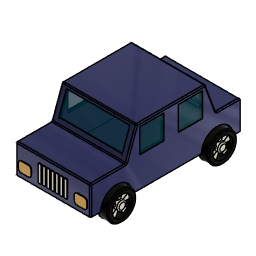
P7 (Autodesk Fusion 360 design; units mm, degrees)
Autodesk Fusion 360 part; units mm, degrees
note: some values were not read from the file. Chosen so that the rebuilt part matches the saved one: which bodies a step acts on. Set by a fixed rule: which sketch regions a step uses.
sketch "Sketch1" plane through (0, 0, 0) normal (1, 0, 0) x (0, 1, 0)
  line L0 (-140, 0) -> (120, 0)
  line L1 (120, 0) -> (120, 50)
  line L2 (120, 50) -> (78.1985, 50)
  line L3 (78.1985, 50) -> (60, 100)
  line L4 (60, 100) -> (-60, 100)
  line L5 (-60, 100) -> (-78.1985, 50)
  line L6 (-78.1985, 50) -> (-140, 50)
  line L7 (-140, 50) -> (-140, 0)
  line L8 (0, 0) -> (0, 100) construction
  dimension "d1" = 120
  dimension "d2" = 50
  dimension "d3" = 100
  dimension "d4" = 120
  dimension "d5" = 260
  dimension "d6" = 110
  dimension "d7" = 110
  constraint horizontal L0
  constraint perpendicular L1 L2
  constraint coincident L8.start origin
  constraint midpoint L4 L8.end
  constraint perpendicular L4 L8
  constraint symmetric L3 L5 L8
  constraint collinear L2 L6
  constraint vertical L7
  constraint perpendicular L6 L7
  constraint coincident L8.start L0
  measures "d1" distance of L3.end L4.end
  measures "d2" distance of L0.end L1.end
  measures "d3" distance of L0 L3.end
  measures "d4" horizontal distance of L8.start L0.end
  measures "d5" distance of L0.start L0.end
  measures "d6" angle of L5 L6
  measures "d7" angle of L2 L3
extrude "Extrude1" add sketch "Sketch1" along normal mid plane 130 makes body 1
shell "Shell1" thickness 5 removed faces 0 bodies 1
sketch "Sketch2" plane through (65, 0, 0) normal (1, 0, 0) x (0, 1, 0)
  line L0 (-140, 50) -> (-140, 0)
  line L1 (-140, 0) -> (120, 0)
  line L2 (120, 0) -> (120, 50)
  line L3 (120, 50) -> (78.1985, 50)
  line L4 (78.1985, 50) -> (60, 100)
  line L5 (60, 100) -> (-60, 100)
  line L6 (-60, 100) -> (-78.1985, 50)
  line L7 (-78.1985, 50) -> (-140, 50)
  line L8 (0, 0) -> (0, 100) construction
  line L9 (-12.5, 94) -> (-54.5, 94)
  line L10 (-54.5, 94) -> (-54.5, 52)
  line L11 (-54.5, 52) -> (-12.5, 52)
  line L12 (-12.5, 52) -> (-12.5, 94)
  line L13 (12.5, 52) -> (12.5, 94)
  line L14 (12.5, 94) -> (54.5, 94)
  line L15 (54.5, 94) -> (54.5, 52)
  line L16 (54.5, 52) -> (12.5, 52)
  dimension "d16" = 42
  dimension "d17" = 42
  dimension "d18" = 12.5
  dimension "d19" = 6
  constraint coincident L8.start origin
  constraint midpoint L5 L8.end
  constraint horizontal L9
  constraint vertical L10
  constraint horizontal L11
  constraint vertical L12
  constraint symmetric L9.start L8 L13.end
  constraint symmetric L8 L9.end L14.end
  constraint symmetric L8 L10.end L15.end
  constraint symmetric L8 L11.end L13.start
  measures "d16" distance of L9.start L9.end
  measures "d17" distance of L9.start L11.end
  measures "d18" horizontal distance of L9.start L8.end
  measures "d19" vertical distance of L5.end L9.end
extrude "Extrude2" cut sketch "Sketch2" against normal blind 130 contours L9 L10 L11 L12 | L13 L14 L15 L16 bodies 1
sketch "Sketch3" plane through (0, 0, 0) normal (0, 1, 0) x (1, 0, 0)
  line L0 (55, -95) -> (-55, -95)
  line L1 (-55, -95) -> (-55, -55)
  line L2 (-55, -55) -> (55, -55)
  line L3 (55, -55) -> (55, -95)
  line L4 (-65, -100) -> (65, -100)
  line L5 (0, 0) -> (0, -100) construction
  dimension "d24" = 5
  dimension "d25" = 40
  dimension "d26" = 110
  constraint horizontal L0
  constraint vertical L1
  constraint horizontal L2
  constraint vertical L3
  constraint coincident L5.start origin
  constraint midpoint L4 L5.end
  constraint symmetric L1 L3 L5
  measures "d24" distance of L0.end L4
  measures "d25" distance of L0.end L1.end
  measures "d26" distance of L0.start L0.end
extrude "Extrude3" cut sketch "Sketch3" along normal mid plane 150 bodies 1
sketch "Sketch4" plane through (65, 0, 0) normal (1, 0, 0) x (0, 1, 0)
  line L0 (-54.5, 94) -> (-12.5, 94)
  line L1 (-12.5, 94) -> (-12.5, 52)
  line L2 (-12.5, 52) -> (-54.5, 52)
  line L3 (-54.5, 52) -> (-54.5, 94)
  line L4 (12.5, 94) -> (54.5, 94)
  line L5 (54.5, 94) -> (54.5, 52)
  line L6 (54.5, 52) -> (12.5, 52)
  line L7 (12.5, 52) -> (12.5, 94)
  line L8 (-140, 50) -> (-140, 0)
  line L9 (-140, 0) -> (120, 0)
  line L10 (120, 0) -> (120, 50)
  line L11 (120, 50) -> (78.1985, 50)
  line L12 (78.1985, 50) -> (60, 100)
  line L13 (60, 100) -> (-60, 100)
  line L14 (-60, 100) -> (-78.1985, 50)
  line L15 (-78.1985, 50) -> (-140, 50)
  line L16 (-54.5, 94) -> (-12.5, 94)
  line L17 (-12.5, 94) -> (-12.5, 52)
  line L18 (-12.5, 52) -> (-54.5, 52)
  line L19 (-54.5, 52) -> (-54.5, 94)
  line L20 (12.5, 94) -> (54.5, 94)
  line L21 (54.5, 94) -> (54.5, 52)
  line L22 (54.5, 52) -> (12.5, 52)
  line L23 (12.5, 52) -> (12.5, 94)
  constraint horizontal L16
  constraint vertical L17
  constraint horizontal L18
  constraint vertical L19
  constraint coincident L1.end L2.start
  constraint coincident L0.start L3.end
  constraint horizontal L20
  constraint vertical L21
  constraint horizontal L22
  constraint vertical L23
  constraint coincident L5.end L6.start
  constraint coincident L4.start L7.end
extrude "Extrude4" add sketch "Sketch4" against normal blind 2 separate body contours L0 L1 L2 L3 L16 L17 L18 L19 | L4 L5 L6 L7 L20 L21 L22 L23 makes body 2 at (65, -40.5, 80) makes body 3 at (65, 40.5, 66)
mirror "Mirror1" about plane through (0, 0, 0) normal (1, 0, 0) of bodies 2 3 makes body 4 at (-65, -40.5, 80) makes body 5 at (-65, 40.5, 66)
sketch "Sketch5" plane through (0, -85.1207, 30.9814) normal (0, -0.939693, 0.34202) x (1, 0, 0)
  line L0 (55, 29.591) -> (-55, 29.591)
  line L1 (-55, 29.591) -> (-55, 68.1272)
  line L2 (-55, 68.1272) -> (55, 68.1272)
  line L3 (55, 68.1272) -> (55, 29.591)
  line L4 (-65, 20.2392) -> (65, 20.2392)
  line L5 (65, 20.2392) -> (65, 73.4481)
  line L6 (65, 73.4481) -> (-65, 73.4481)
  line L7 (-65, 73.4481) -> (-65, 20.2392)
  line L8 (-55, 29.591) -> (55, 29.591)
  line L9 (55, 29.591) -> (55, 68.1272)
  line L10 (55, 68.1272) -> (-55, 68.1272)
  line L11 (-55, 68.1272) -> (-55, 29.591)
  constraint horizontal L8
  constraint vertical L9
  constraint horizontal L10
  constraint vertical L11
  constraint coincident L2.end L3.start
  constraint coincident L0.end L1.start
extrude "Extrude5" add sketch "Sketch5" against normal blind 2 separate body contours L0 L1 L2 L3 L8 L9 L10 L11 makes body 6
mirror "Mirror2" about plane through (0, 0, 0) normal (0, 1, 0) of bodies 6 makes body 7
sketch "Sketch6" plane through (0, -140, 0) normal (0, -1, 0) x (1, 0, 0)
  line L0 (-65, 0) -> (65, 0)
  line L1 (65, 0) -> (65, 50)
  line L2 (65, 50) -> (-65, 50)
  line L3 (-65, 50) -> (-65, 0)
  line L4 (0, 0) -> (0, 50) construction
  line L5 (-54.5, 26) -> (-42.5, 26)
  line L6 (-37.5, 21) -> (-37.5, 13)
  line L7 (-42.5, 8) -> (-54.5, 8)
  line L8 (-59.5, 13) -> (-59.5, 21)
  arc A0 (-54.5, 26) -> (-59.5, 21) centre (-54.5, 21) ccw
  arc A1 (-37.5, 21) -> (-42.5, 26) centre (-42.5, 21) ccw
  arc A2 (-59.5, 13) -> (-54.5, 8) centre (-54.5, 13) ccw
  arc A3 (-42.5, 8) -> (-37.5, 13) centre (-42.5, 13) ccw
  arc A4 (42.5, 26) -> (37.5, 21) centre (42.5, 21) ccw
  line L9 (54.5, 26) -> (42.5, 26)
  arc A5 (59.5, 21) -> (54.5, 26) centre (54.5, 21) ccw
  line L10 (59.5, 13) -> (59.5, 21)
  arc A6 (54.5, 8) -> (59.5, 13) centre (54.5, 13) ccw
  line L11 (42.5, 8) -> (54.5, 8)
  arc A7 (37.5, 13) -> (42.5, 8) centre (42.5, 13) ccw
  line L12 (37.5, 21) -> (37.5, 13)
  dimension "d37" = 5
  dimension "d38" = 5
  dimension "d39" = 5
  dimension "d40" = 5
  dimension "d41" = 18
  dimension "d42" = 22
  dimension "d43" = 8
  dimension "d44" = 37.5
  constraint coincident L4.start origin
  constraint midpoint L2 L4.end
  constraint horizontal L5
  constraint vertical L6
  constraint horizontal L7
  constraint vertical L8
  constraint tangent L8 A0
  constraint tangent L5 A0
  constraint tangent L5 A1
  constraint tangent L6 A1
  constraint tangent L8 A2
  constraint tangent L7 A2
  constraint tangent L7 A3
  constraint tangent L6 A3
  constraint symmetric L4 L8.end A5.start
  constraint symmetric L4 L5.start L9.start
  constraint symmetric L4 A0 A5
  constraint symmetric L4 L5.end A4.start
  constraint symmetric L4 L6.start A4.end
  constraint symmetric L4 A1 A4
  constraint symmetric L4 L8.start L10.start
  constraint symmetric L4 L7.end A6.start
  constraint symmetric L4 A2 A6
  constraint symmetric L4 L7.start L11.start
  constraint symmetric L4 L6.end A7.start
  constraint symmetric L4 A3 A7
  measures "d37" radius of A0
  measures "d38" radius of A1
  measures "d39" radius of A2
  measures "d40" radius of A3
  measures "d41" distance of L5 L7
  measures "d42" distance of L6 L8
  measures "d43" distance of L0 L7
  measures "d44" distance of L4 L6
extrude "Extrude6" add sketch "Sketch6" along normal blind 1 contours L5 L6 L7 L8 A0 A1 A2 A3 | A4 L9 A5 L10 A6 L11 A7 L12 bodies 1
sketch "Sketch7" plane through (0, 120, 0) normal (0, 1, 0) x (-1, 0, 0)
  line L0 (65, 50) -> (-65, 50)
  line L1 (-65, 50) -> (-65, 0)
  line L2 (-65, 0) -> (65, 0)
  line L3 (65, 0) -> (65, 50)
  line L4 (-54.5, 26) -> (-42.5, 26)
  line L5 (-37.5, 21) -> (-37.5, 13)
  line L6 (-42.5, 8) -> (-54.5, 8)
  line L7 (-59.5, 13) -> (-59.5, 21)
  arc A0 (-54.5, 26) -> (-59.5, 21) centre (-54.5, 21) ccw
  arc A1 (-59.5, 13) -> (-54.5, 8) centre (-54.5, 13) ccw
  arc A2 (-42.5, 8) -> (-37.5, 13) centre (-42.5, 13) ccw
  arc A3 (-37.5, 21) -> (-42.5, 26) centre (-42.5, 21) ccw
  line L8 (0, 0) -> (0, 50) construction
  arc A4 (42.5, 26) -> (37.5, 21) centre (42.5, 21) ccw
  line L9 (54.5, 26) -> (42.5, 26)
  arc A5 (59.5, 21) -> (54.5, 26) centre (54.5, 21) ccw
  line L10 (59.5, 13) -> (59.5, 21)
  arc A6 (54.5, 8) -> (59.5, 13) centre (54.5, 13) ccw
  line L11 (42.5, 8) -> (54.5, 8)
  arc A7 (37.5, 13) -> (42.5, 8) centre (42.5, 13) ccw
  line L12 (37.5, 21) -> (37.5, 13)
  dimension "d47" = 5
  dimension "d48" = 22
  dimension "d49" = 37.5
  dimension "d50" = 18
  dimension "d51" = 8
  constraint horizontal L4
  constraint vertical L5
  constraint horizontal L6
  constraint vertical L7
  constraint tangent L4 A0
  constraint tangent L7 A0
  constraint tangent L6 A1
  constraint tangent L7 A1
  constraint equal A0 A1
  constraint tangent L6 A2
  constraint tangent L5 A2
  constraint equal A0 A2
  constraint tangent L4 A3
  constraint tangent L5 A3
  constraint equal A0 A3
  constraint coincident L8.start origin
  constraint midpoint L0 L8.end
  constraint symmetric L4.start L8 L9.start
  constraint symmetric L7.end L8 A5.start
  constraint symmetric A0 L8 A5
  constraint symmetric L6.end L8 A6.start
  constraint symmetric L7.start L8 L10.start
  constraint symmetric A1 L8 A6
  constraint symmetric L6.start L8 L11.start
  constraint symmetric L5.end L8 A7.start
  constraint symmetric A2 L8 A7
  constraint symmetric L4.end L8 A4.start
  constraint symmetric L5.start L8 A4.end
  constraint symmetric A3 L8 A4
  measures "d47" radius of A0
  measures "d48" distance of L5 L7
  measures "d49" distance of L5 L8
  measures "d50" distance of L4 L6
  measures "d51" distance of L2 L6
extrude "Extrude7" add sketch "Sketch7" along normal blind 1 contours L4 L5 L6 L7 A0 A1 A2 A3 | A4 L9 A5 L10 A6 L11 A7 L12 bodies 1
sketch "Sketch8" plane through (0, -140, 0) normal (0, -1, 0) x (1, 0, 0)
  arc A0 (42.5, 26) -> (37.5, 21) centre (42.5, 21) ccw
  line L0 (42.5, 26) -> (54.5, 26)
  arc A1 (59.5, 21) -> (54.5, 26) centre (54.5, 21) ccw
  line L1 (59.5, 21) -> (59.5, 13)
  arc A2 (54.5, 8) -> (59.5, 13) centre (54.5, 13) ccw
  line L2 (54.5, 8) -> (42.5, 8)
  arc A3 (37.5, 13) -> (42.5, 8) centre (42.5, 13) ccw
  line L3 (37.5, 13) -> (37.5, 21)
  line L4 (-59.5, 13) -> (-59.5, 21)
  arc A4 (-54.5, 26) -> (-59.5, 21) centre (-54.5, 21) ccw
  line L5 (-54.5, 26) -> (-42.5, 26)
  arc A5 (-37.5, 21) -> (-42.5, 26) centre (-42.5, 21) ccw
  line L6 (-37.5, 21) -> (-37.5, 13)
  arc A6 (-42.5, 8) -> (-37.5, 13) centre (-42.5, 13) ccw
  line L7 (-42.5, 8) -> (-54.5, 8)
  arc A7 (-59.5, 13) -> (-54.5, 8) centre (-54.5, 13) ccw
  line L8 (-65, 0) -> (65, 0)
  line L9 (65, 0) -> (65, 50)
  line L10 (65, 50) -> (-65, 50)
  line L11 (-65, 50) -> (-65, 0)
  line L12 (-25, 38) -> (-20, 38)
  line L13 (-20, 38) -> (-20, 8)
  line L14 (-20, 8) -> (-25, 8)
  line L15 (-25, 8) -> (-25, 38)
  line L16 (0, 0) -> (0, 50) construction
  line L17 (-17.5, 8) -> (-17.5, 38)
  line L18 (-12.5, 38) -> (-12.5, 8)
  line L19 (-17.5, 38) -> (-12.5, 38)
  line L20 (-12.5, 8) -> (-17.5, 8)
  line L21 (-10, 8) -> (-10, 38)
  line L22 (-5, 38) -> (-5, 8)
  line L23 (-10, 38) -> (-5, 38)
  line L24 (-5, 8) -> (-10, 8)
  line L25 (-2.5, 8) -> (-2.5, 38)
  line L26 (2.5, 38) -> (2.5, 8)
  line L27 (-2.5, 38) -> (2.5, 38)
  line L28 (2.5, 8) -> (-2.5, 8)
  line L29 (5, 8) -> (5, 38)
  line L30 (10, 38) -> (10, 8)
  line L31 (5, 38) -> (10, 38)
  line L32 (10, 8) -> (5, 8)
  line L33 (12.5, 8) -> (12.5, 38)
  line L34 (17.5, 38) -> (17.5, 8)
  line L35 (12.5, 38) -> (17.5, 38)
  line L36 (17.5, 8) -> (12.5, 8)
  line L37 (20, 8) -> (20, 38)
  line L38 (25, 38) -> (25, 8)
  line L39 (20, 38) -> (25, 38)
  line L40 (25, 8) -> (20, 8)
  dimension "d54" = 5
  dimension "d55" = 30
  dimension "d56" = 8
  dimension "d58" = 25
  dimension "d61" = 7.5
  dimension "d62" = 0
  constraint horizontal L12
  constraint vertical L13
  constraint horizontal L14
  constraint vertical L15
  constraint coincident L16.start origin
  constraint midpoint L10 L16.end
  measures "d54" distance of L12.start L12.end
  measures "d55" distance of L12.start L14.end
  measures "d56" distance of L8 L14.end
  measures "d58" distance of L15 L16
extrude "Extrude8" add sketch "Sketch8" along normal blind 1 separate body contours L12 L13 L14 L15 | L17 L18 L19 L20 | L21 L22 L23 L24 | L25 L26 L27 L28 | L29 L30 L31 L32 | L33 L34 L35 L36 | L37 L38 L39 L40 makes body 8 at (6.6667, -140, 28) makes body 9 at (-23.3333, -140, 28) makes body 10 at (-0.8333, -140, 28) makes body 11 at (14.1667, -140, 28) makes body 12 at (-15.8333, -140, 28) makes body 13 at (-8.3333, -140, 28) makes body 14 at (21.6667, -140, 28)
sketch "Sketch9" plane through (65, 0, 0) normal (1, 0, 0) x (0, 1, 0)
  line L0 (-54.5, 94) -> (-12.5, 94)
  line L1 (-12.5, 94) -> (-12.5, 52)
  line L2 (-12.5, 52) -> (-54.5, 52)
  line L3 (-54.5, 52) -> (-54.5, 94)
  line L4 (12.5, 94) -> (54.5, 94)
  line L5 (54.5, 94) -> (54.5, 52)
  line L6 (54.5, 52) -> (12.5, 52)
  line L7 (12.5, 52) -> (12.5, 94)
  line L8 (-140, 50) -> (-140, 0)
  line L9 (-140, 0) -> (120, 0)
  line L10 (120, 0) -> (120, 50)
  line L11 (120, 50) -> (78.1985, 50)
  line L12 (78.1985, 50) -> (60, 100)
  line L13 (60, 100) -> (-60, 100)
  line L14 (-60, 100) -> (-78.1985, 50)
  line L15 (-78.1985, 50) -> (-140, 50)
  circle A0 centre (-95, 0) radius 27.5
  circle A1 centre (80, 0) radius 27.5
  dimension "d65" = 55
  dimension "d66" = 55
  dimension "d67" = 45
  dimension "d69" = 175
  constraint coincident L9 A0.centre
  constraint coincident L9 A1.centre
  measures "d65" diameter of A0
  measures "d66" diameter of A1
  measures "d67" distance of L8.end A0.centre
  measures "d69" distance of A0.centre A1.centre
extrude "Extrude9" cut sketch "Sketch9" against normal blind 15 contours L9 A0 | L9 A0 | L9 A1 | L9 A1 bodies 1
mirror "Mirror3" about plane through (0, 0, 0) normal (1, 0, 0) of "Extrude9"
sketch "Sketch10" plane through (65, 0, 0) normal (1, 0, 0) x (0, 1, 0)
  arc A0 (-67.5, 0) -> (-122.5, 0) centre (-95, 0) ccw
  line L0 (-67.5, 0) -> (52.5, 0)
  arc A1 (107.5, 0) -> (52.5, 0) centre (80, 0) ccw
  line L1 (107.5, 0) -> (120, 0)
  line L2 (120, 0) -> (120, 50)
  line L3 (120, 50) -> (78.1985, 50)
  line L4 (78.1985, 50) -> (60, 100)
  line L5 (60, 100) -> (-60, 100)
  line L6 (-60, 100) -> (-78.1985, 50)
  line L7 (-78.1985, 50) -> (-140, 50)
  line L8 (-140, 50) -> (-140, 0)
  line L9 (-140, 0) -> (-122.5, 0)
  line L10 (-54.5, 94) -> (-12.5, 94)
  line L11 (-12.5, 94) -> (-12.5, 52)
  line L12 (-12.5, 52) -> (-54.5, 52)
  line L13 (-54.5, 52) -> (-54.5, 94)
  line L14 (12.5, 94) -> (54.5, 94)
  line L15 (54.5, 94) -> (54.5, 52)
  line L16 (54.5, 52) -> (12.5, 52)
  line L17 (12.5, 52) -> (12.5, 94)
  circle A2 centre (-95, 0) radius 17.5
  circle A3 centre (-95, 0) radius 7.5
  circle A4 centre (-95, 0) radius 25
  circle A5 centre (80, 0) radius 25
  circle A6 centre (80, 0) radius 17.5
  circle A7 centre (80, 0) radius 7.5
  dimension "d74" = 35
  dimension "d75" = 15
  dimension "d76" = 50
  dimension "d77" = 50
  dimension "d78" = 35
  dimension "d79" = 15
  constraint concentric A0 A2
  constraint concentric A0 A3
  constraint concentric A3 A4
  constraint concentric A1 A5
  constraint concentric A1 A6
  constraint concentric A6 A7
  measures "d74" diameter of A2
  measures "d75" diameter of A3
  measures "d76" diameter of A4
  measures "d77" diameter of A5
  measures "d78" diameter of A6
  measures "d79" diameter of A7
extrude "Extrude10" add sketch "Sketch10" along normal mid plane 20 separate body contours A3 | A4 | A5 | A7 makes body 15 at (71.6667, -87.5093, -0.3738) makes body 16 at (71.6667, 104.9689, -1.2461) makes body 17 at (71.6667, -70.0311, -1.2461) makes body 18 at (71.6667, 87.4907, -0.3738)
sketch "Sketch11" plane through (65, 0, 0) normal (1, 0, 0) x (0, 1, 0)
  arc A0 (-67.5, 0) -> (-122.5, 0) centre (-95, 0) ccw
  line L0 (-67.5, 0) -> (52.5, 0)
  arc A1 (107.5, 0) -> (52.5, 0) centre (80, 0) ccw
  line L1 (107.5, 0) -> (120, 0)
  line L2 (120, 0) -> (120, 50)
  line L3 (120, 50) -> (78.1985, 50)
  line L4 (78.1985, 50) -> (60, 100)
  line L5 (60, 100) -> (-60, 100)
  line L6 (-60, 100) -> (-78.1985, 50)
  line L7 (-78.1985, 50) -> (-140, 50)
  line L8 (-140, 50) -> (-140, 0)
  line L9 (-140, 0) -> (-122.5, 0)
  line L10 (-54.5, 94) -> (-12.5, 94)
  line L11 (-12.5, 94) -> (-12.5, 52)
  line L12 (-12.5, 52) -> (-54.5, 52)
  line L13 (-54.5, 52) -> (-54.5, 94)
  line L14 (12.5, 94) -> (54.5, 94)
  line L15 (54.5, 94) -> (54.5, 52)
  line L16 (54.5, 52) -> (12.5, 52)
  line L17 (12.5, 52) -> (12.5, 94)
  line L18 (-95, 0) -> (-95, 25.1648) construction
  line L19 (-92.6885, 7.1349) -> (-90.0989, 16.7997)
  line L20 (-97.3115, 7.1349) -> (-99.9011, 16.7997)
  circle A2 centre (-95, 0) radius 17.5
  circle A3 centre (-95, 0) radius 7.5
  line L21 (-101.0714, 4.4031) -> (-109.4629, 9.8526)
  line L22 (-102.5, 0.0065) -> (-112.492, 0.5301)
  line L23 (-101.0638, -4.4136) -> (-108.8397, -10.7104)
  line L24 (-97.3238, -7.1309) -> (-100.9095, -16.472)
  line L25 (-92.6762, -7.1309) -> (-89.0905, -16.472)
  line L26 (-88.9362, -4.4136) -> (-81.1603, -10.7104)
  line L27 (-87.5, 0.0065) -> (-77.508, 0.5301)
  line L28 (-88.9286, 4.4031) -> (-80.5371, 9.8526)
  arc A4 (-77.508, 0.5301) -> (-80.5371, 9.8526) centre (-95, 0) ccw
  arc A5 (-89.0905, -16.472) -> (-81.1603, -10.7104) centre (-95, 0) ccw
  arc A6 (-108.8397, -10.7104) -> (-100.9095, -16.472) centre (-95, 0) ccw
  arc A7 (-90.0989, 16.7997) -> (-99.9011, 16.7997) centre (-95, 0) ccw
  arc A8 (-109.4629, 9.8526) -> (-112.492, 0.5301) centre (-95, 0) ccw
  dimension "d82" = 30
  dimension "d84" = 360
  constraint coincident A0.centre L18.start
  constraint vertical L18
  constraint symmetric L18 L19 L20
  constraint coincident L19.end A2
  constraint coincident L19.start A3
  constraint coincident L20.start A3
  constraint coincident L20.end A2
  constraint concentric A2 A7
  constraint coincident L27.end A7
  constraint concentric A4 A7
  constraint concentric A5 A7
  constraint concentric A6 A7
  constraint concentric A7 A8
  measures "d82" angle of L19 L20
extrude "Extrude11" add sketch "Sketch11" along normal mid plane 10 separate body contours L19 L20 A2 A3 A7 | A2 A3 L27 L28 A4 | A2 A3 L21 L22 A8 | A2 A3 L25 L26 A5 | A2 A3 L23 L24 A6 makes body 19 at (66.6667, -98.519, -10.2446) makes body 20 at (66.6667, -105.8307, 0.181) makes body 21 at (66.6667, -83.7523, -8.6115) makes body 22 at (63.3333, -98.1747, 10.3565) makes body 23 at (66.6667, -83.3342, 8.0361)
pattern_linear "R-Pattern1" count 2 spacing 175 along (0, 1, 0) of bodies 23 22 20 19 21 makes body 24 at (66.6667, 76.481, -10.2446) makes body 25 at (66.6667, 69.1693, 0.181) makes body 26 at (66.6667, 91.2477, -8.6115) makes body 27 at (63.3333, 76.8253, 10.3565) makes body 28 at (66.6667, 91.6658, 8.0361)
fillet "Fillet1" radius 2 8 edges at (75, -101.9925, -2.7121) (55, -101.9925, 2.7121) (75, 56.6918, -9.0404) (55, 56.6918, 9.0404) (75, -118.3082, -9.0404) (55, -118.3082, 9.0404) (75, 73.0075, -2.7121) (55, 73.0075, 2.7121) on bodies 15 16 17 18
mirror "Mirror4" about plane through (0, 0, 0) normal (1, 0, 0) of bodies 17 23 22 20 19 21 15 16 27 25 18 28 26 24 makes body 29 at (-67.6667, -87.5373, -0.7468) makes body 30 at (-67.6667, 104.8758, -2.4892) makes body 31 at (-67.6667, -70.1242, -2.4892) makes body 32 at (-67.6667, 87.4627, -0.7468) makes body 33 at (-66.6667, -98.519, -10.2446) makes body 34 at (-66.6667, -105.8307, 0.181) makes body 35 at (-66.6667, -83.7523, -8.6115) makes body 36 at (-63.3333, -98.1747, 10.3565) makes body 37 at (-66.6667, -83.3342, 8.0361) makes body 38 at (-66.6667, 76.481, -10.2446) makes body 39 at (-66.6667, 69.1693, 0.181) makes body 40 at (-66.6667, 91.2477, -8.6115) makes body 41 at (-63.3333, 76.8253, 10.3565) makes body 42 at (-66.6667, 91.6658, 8.0361)
fillet "Fillet2" radius 2 19 edges at (-65, -140, 25) (-65, -109.0993, 50) (0, -140, 50) (65, -140, 25) (65, -109.0993, 50) (65, -69.0993, 75) (0, -60, 100) (-65, -69.0993, 75) (65, 0, 100) (-65, 0, 100) (0, 60, 100) (65, 69.0993, 75) (65, 99.0993, 50) (-65, 69.0993, 75) (-65, 99.0993, 50) (-65, 120, 25) (0, 120, 50) (0, 78.1985, 50) (0, -78.1985, 50) on bodies 1
